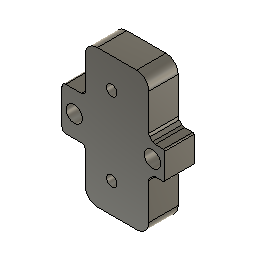
model (Autodesk Fusion 360 design; units mm, degrees)
Autodesk Fusion 360 part; units mm, degrees
sketch "Sketch1" plane through (0, 0, 0) normal (0, 1, 0) x (1, 0, 0)
  line L0 (0, 0) -> (26, 0)
  line L1 (26, 0) -> (26, -56.5)
  line L2 (26, -56.5) -> (0, -56.5)
  line L3 (0, -56.5) -> (0, 0)
  line L4 (0, -37) -> (-9.5, -37)
  line L5 (-9.5, -37) -> (-9.5, -19.5)
  line L6 (-9.5, -19.5) -> (0, -19.5)
  line L7 (-9.5, -28.25) -> (0, -28.25) construction
  line L8 (26, -34) -> (32.5, -34)
  line L9 (32.5, -34) -> (32.5, -22.5)
  line L10 (32.5, -22.5) -> (26, -22.5)
  line L11 (26, -28.25) -> (32.5, -28.25) construction
  circle A0 centre (10.85, -44.25) radius 2.15
  circle A1 centre (10.85, -12.25) radius 2.15
  line L12 (10.85, -44.25) -> (10.85, -12.25) construction
  line L13 (0, -28.25) -> (10.85, -28.25) construction
  line L14 (8.7, -44.25) -> (10.85, -44.25) construction
  point P0 (8.7, -44.25)
  dimension "d2" = 26
  dimension "d3" = 56.5
  dimension "d4" = 9.5
  dimension "d5" = 17.5
  dimension "d6" = 6.5
  dimension "d7" = 11.5
  dimension "d8" = 32
  dimension "d9" = 4.3
  dimension "d10" = 8.7
  constraint horizontal L0
  constraint vertical L1
  constraint horizontal L2
  constraint vertical L3
  constraint coincident L0.start L3.end
  constraint coincident L3 L4.start
  constraint coincident L3 L6.end
  constraint vertical L5
  constraint horizontal L6
  constraint horizontal L4
  constraint midpoint L5 L7.start
  constraint midpoint L3 L7.end
  constraint horizontal L7
  constraint coincident L1 L8.start
  constraint coincident L1 L10.end
  constraint horizontal L8
  constraint vertical L9
  constraint horizontal L10
  constraint midpoint L1 L11.start
  constraint midpoint L9 L11.end
  constraint horizontal L11
  constraint coincident A0.centre L12.start
  constraint coincident A1.centre L12.end
  constraint vertical L12
  constraint midpoint L12 L13.end
  constraint horizontal L13
  constraint equal A0 A1
  constraint coincident A0 P0
  constraint coincident P0 L14.start
  constraint horizontal L14
  measures "d2" distance of L1.end L2.end
  measures "d3" distance of L0.end L1.end
  measures "d4" horizontal distance of L2.end L4.end
  measures "d5" distance of L4.end L5.end
  measures "d6" distance of L8.start L8.end
  measures "d7" distance of L8.end L9.end
  measures "d8" distance of A0.centre A1.centre
  measures "d9" diameter of A1
  measures "d10" horizontal distance of L2.end P0
extrude "Extrude1" add sketch "Sketch1" along normal blind 12
sketch "Sketch2" plane through (0, 0, 0) normal (0, -1, 0) x (1, 0, 0)
  circle A0 centre (10.85, 12.25) radius 2.15
  circle A1 centre (10.85, 44.25) radius 2.15
  line L0 (32.5, 34) -> (26, 34)
  line L1 (26, 34) -> (26, 56.5)
  line L2 (26, 56.5) -> (0, 56.5)
  line L3 (0, 56.5) -> (0, 37)
  line L4 (0, 37) -> (-9.5, 37)
  line L5 (-9.5, 37) -> (-9.5, 19.5)
  line L6 (-9.5, 19.5) -> (0, 19.5)
  line L7 (0, 19.5) -> (0, 0)
  line L8 (0, 0) -> (26, 0)
  line L9 (26, 0) -> (26, 22.5)
  line L10 (26, 22.5) -> (32.5, 22.5)
  line L11 (32.5, 22.5) -> (32.5, 34)
  line L12 (-9.5, 28.25) -> (32.5, 28.25) construction
  circle A2 centre (-4.5, 28.25) radius 3.3
  circle A3 centre (-4.5, 28.25) radius 1.75
  circle A4 centre (27.5, 28.25) radius 1.75
  circle A5 centre (27.5, 28.25) radius 3.3
  dimension "d20" = 3.5
  dimension "d21" = 6.6
  dimension "d22" = 5
  dimension "d23" = 5
  constraint midpoint L5 L12.start
  constraint midpoint L11 L12.end
  constraint coincident L12 A2.centre
  constraint concentric A2 A3
  constraint coincident L12 A4.centre
  constraint concentric A4 A5
  constraint equal A3 A4
  constraint equal A2 A5
  measures "d20" diameter of A3
  measures "d21" diameter of A2
  measures "d22" horizontal distance of L0.start A4.centre
  measures "d23" horizontal distance of L4.end A2.centre
extrude "Extrude2" cut sketch "Sketch2" against normal up to surface (12 mm away) contours A3 | A4
extrude "Extrude3" cut sketch "Sketch2" against normal up to surface (9 mm away) contours A2 | A5
chamfer "Chamfer2" distance 1.55 angle 45 2 edges at (-6.1316, 9, 27.6172) (25.8684, 9, 27.6172)
chamfer "Chamfer1" distance 2 angle 45 2 edges at (26, 6, 34) (26, 6, 22.5)
fillet "Fillet1" radius 1.5 8 edges at (0, 6, 37) (0, 6, 19.5) (26, 6, 36) (28, 6, 34) (26, 6, 20.5) (28, 6, 22.5) (-9.5, 6, 37) (-9.5, 6, 19.5)
fillet "Fillet2" radius 5 4 edges at (26, 6, 0) (0, 6, 56.5) (26, 6, 56.5) (0, 6, 0)
fillet "Fillet3" radius 0.5 2 edges at (32.5, 6, 34) (32.5, 6, 22.5)
equation "d11 = thickness"
equation "thickness = 12 mm"
